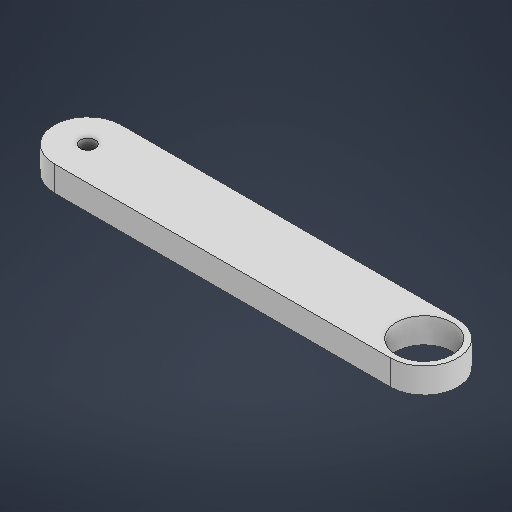
# Autodesk Inventor part: Uleg
Saved by Autodesk Inventor 2026.2 (Build 302298010, 298A)
## iProperties
Created: 2026-05-06
Part Number: Uleg
Material: Generic
Document SubType Name: Modeling
Designer: Martina
Density: 1 g/cm^3
Appearance: Default
Author: Martina
Autodesk Inventor part; units mm, degrees
ref_plane "YZ Plane" through (0, 0, 0) normal (1, 0, 0) x (0, 1, 0)
ref_plane "XZ Plane" through (0, 0, 0) normal (0, 1, 0) x (-1, 0, 0)
ref_plane "XY Plane" through (0, 0, 0) normal (0, 0, 1) x (1, 0, 0)
sketch "Sketch1" plane through (0, 0, 0) normal (0, 1, 0) x (-1, 0, 0)
  arc A0 (-39.909, 7.7247) -> (-39.909, -6.6753) centre (-39.909, 0.5247) ccw
  arc A1 (32.091, -6.6753) -> (32.091, 7.7247) centre (32.091, 0.5247) ccw
  line L0 (32.091, -6.6753) -> (-39.909, -6.6753)
  line L1 (-39.909, 7.7247) -> (32.091, 7.7247)
  circle A2 centre (32.091, 0.5247) radius 1.6
  circle A3 centre (-39.909, 0.5247) radius 6
  point P0 (-47.109, 0.5247)
  point P1 (39.291, 0.5247)
  dimension "d34" = 14.4
  dimension "d35" = 86.4
  dimension "d36" = 3.2
  dimension "d37" = 12
  dimension "d38" = 7.2
  constraints: 6 point on circle, 4 centre point, 4 end point, 3 tangent, 2 coincident, 1 parallel
  measures "d34" diameter of A1
  measures "d35" distance of point (-47.109, 0.525) point (39.291, 0.525)
  measures "d36" diameter of A2
  measures "d37" diameter of A3
  measures "d38" radius of A1
extrude "Extrusion2" add sketch "Sketch1" along normal mid plane 5.4
body "Solid1"
